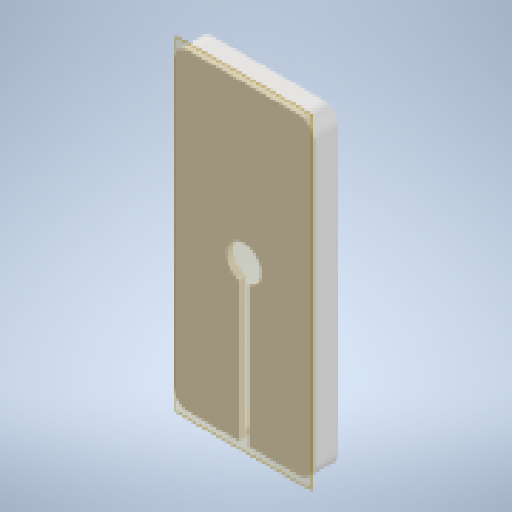
# Autodesk Inventor part: cache_batterie_1
Saved by Autodesk Inventor 2023 (Build 270158000, 158)
## iProperties
Created: 2023-03-28
Part Number: cache_batterie_1
Material: Générique
Document SubType Name: Modeling
Designer: eleves
Density: 1 g/cm^3
Appearance: Par défaut
Author: eleves
Autodesk Inventor part; units mm, degrees
ref_plane "YZ Plane" through (0, 0, 0) normal (1, 0, 0) x (0, 1, 0)
ref_plane "XZ Plane" through (0, 0, 0) normal (0, 1, 0) x (-1, 0, 0)
ref_plane "XY Plane" through (0, 0, 0) normal (0, 0, 1) x (1, 0, 0)
ref_plane "Plan de construction1" through (0, 0, 0) normal (0, 0, 1) x (1, 0, 0)
sketch "Esquisse1" plane through (0, 0, 0) normal (0, 0, 1) x (1, 0, 0)
  arc A0 (0, -82) -> (2, -84) centre (2, -82) ccw construction
  line L0 (2, -84) -> (33, -84) construction
  arc A1 (33, -84) -> (35, -82) centre (33, -82) ccw construction
  line L1 (35, -2) -> (35, -82) construction
  arc A2 (35, -2) -> (33, 0) centre (33, -2) ccw construction
  line L2 (2, 0) -> (33, 0) construction
  arc A3 (2, 0) -> (0, -2) centre (2, -2) ccw construction
  line L3 (0, -2) -> (0, -82) construction
  line L4 (2, -82) -> (33, -82) construction
  line L5 (2, -2) -> (2, -82) construction
  line L6 (2, -2) -> (33, -2) construction
  line L7 (33, -2) -> (33, -82) construction
  arc A4 (33, -84.4) -> (35.4, -82) centre (33, -82) ccw
  line L8 (33, -84.4) -> (2, -84.4)
  arc A5 (-0.4, -82) -> (2, -84.4) centre (2, -82) ccw
  line L9 (-0.4, -82) -> (-0.4, -2)
  arc A6 (2, 0.4) -> (-0.4, -2) centre (2, -2) ccw
  line L10 (2, 0.4) -> (33, 0.4)
  arc A7 (35.4, -2) -> (33, 0.4) centre (33, -2) ccw
  line L11 (35.4, -2) -> (35.4, -82)
  arc A8 (33, -86.4) -> (37.4, -82) centre (33, -82) ccw
  line L12 (33, -86.4) -> (2, -86.4)
  arc A9 (-2.4, -82) -> (2, -86.4) centre (2, -82) ccw
  line L13 (-2.4, -82) -> (-2.4, -2)
  arc A10 (2, 2.4) -> (-2.4, -2) centre (2, -2) ccw
  line L14 (2, 2.4) -> (33, 2.4)
  arc A11 (37.4, -2) -> (33, 2.4) centre (33, -2) ccw
  line L15 (37.4, -2) -> (37.4, -82)
  point P0 (0, 0)
  dimension "d0" = 0.4
  dimension "d1" = 2
  constraints: 16 end point, 16 point on circle, 8 centre point, 14 other
  measures "d0" distance between parallel lines of L1 L11
  measures "d1" distance between parallel lines of L10 L14
extrude "Extrusion1" add sketch "Esquisse1" against normal blind 2 contours L8 A5 L9 A6 L10 A7 L11 A4 | L12 A9 L13 A10 L14 A11 L15 A8
sketch "Esquisse2" plane through (0, 0, -2) normal (0, 0, -1) x (-1, 0, 0)
  line L0 (-33, -86.4) -> (-2, -86.4) projected
  arc A0 (-2, -86.4) -> (2.4, -82) centre (-2, -82) ccw projected
  line L1 (2.4, -82) -> (2.4, -2) projected
  arc A1 (2.4, -2) -> (-2, 2.4) centre (-2, -2) ccw projected
  line L2 (-2, 2.4) -> (-33, 2.4) projected
  arc A2 (-33, 2.4) -> (-37.4, -2) centre (-33, -2) ccw projected
  line L3 (-37.4, -2) -> (-37.4, -82) projected
  arc A3 (-37.4, -82) -> (-33, -86.4) centre (-33, -82) ccw projected
  line L4 (0.4, -2) -> (0.4, -82)
  arc A4 (-2, -84.4) -> (0.4, -82) centre (-2, -82) ccw
  line L5 (-2, -84.4) -> (-33, -84.4)
  arc A5 (-35.4, -82) -> (-33, -84.4) centre (-33, -82) ccw
  line L6 (-35.4, -82) -> (-35.4, -2)
  arc A6 (-33, 0.4) -> (-35.4, -2) centre (-33, -2) ccw
  line L7 (-33, 0.4) -> (-2, 0.4)
  arc A7 (0.4, -2) -> (-2, 0.4) centre (-2, -2) ccw
  point P0 (0, 0)
  dimension "d4" = 2
  constraints: 8 end point, 8 point on circle, 4 centre point, 7 other
  measures "d4" distance between parallel lines of L2 L7
extrude "Extrusion2" add sketch "Esquisse2" along normal blind 5
sketch "Esquisse3" plane through (0, 0, 0) normal (0, 0, 1) x (1, 0, 0)
  line L0 (2, -86.4) -> (33, -86.4) projected
  arc A0 (33, -86.4) -> (37.4, -82) centre (33, -82) ccw projected
  line L1 (37.4, -82) -> (37.4, -2) projected
  arc A1 (37.4, -2) -> (33, 2.4) centre (33, -2) ccw projected
  line L2 (33, 2.4) -> (2, 2.4) projected
  arc A2 (2, 2.4) -> (-2.4, -2) centre (2, -2) ccw projected
  line L3 (-2.4, -2) -> (-2.4, -82) projected
  arc A3 (-2.4, -82) -> (2, -86.4) centre (2, -82) ccw projected
  line L4 (33, -2) -> (2, -82) construction
  line L5 (2, -82) -> (33, -82) construction
  line L6 (2, -84.4) -> (33, -84.4) construction
  line L7 (2, -2) -> (33, -82) construction
  circle A4 centre (17.5, -42) radius 5
  point P0 (0, 0)
  dimension "d7" = 10
  constraints: 6 end point, 1 centre point, 1 midpoint, 1 parallel
  measures "d7" diameter of A4
extrude "Extrusion3" cut sketch "Esquisse3" against normal blind 30.25 contours A4
sketch "Esquisse4" plane through (0, 0, 0) normal (0, 0, 1) x (1, 0, 0)
  circle A0 centre (17.5, -42) radius 5 projected
  line L0 (2, -86.4) -> (33, -86.4) projected
  arc A1 (33, -86.4) -> (37.4, -82) centre (33, -82) ccw projected
  line L1 (37.4, -82) -> (37.4, -2) projected
  arc A2 (37.4, -2) -> (33, 2.4) centre (33, -2) ccw projected
  line L2 (33, 2.4) -> (2, 2.4) projected
  arc A3 (2, 2.4) -> (-2.4, -2) centre (2, -2) ccw projected
  line L3 (-2.4, -2) -> (-2.4, -82) projected
  arc A4 (-2.4, -82) -> (2, -86.4) centre (2, -82) ccw projected
  line L4 (17.5, -42) -> (19.1086, -42)
  line L5 (19.1086, -42) -> (19.1086, -46.7342)
  line L6 (17.5, -42) -> (16.1086, -42)
  line L7 (16.1086, -42) -> (16.1086, -46.8025)
  circle A5 centre (17.5, -42) radius 5 projected
  line L8 (19.1086, -46.7342) -> (19.1086, -86.4)
  line L9 (16.1086, -46.8025) -> (16.1086, -86.4)
  point P0 (0, 0)
  dimension "d11" = 3
  constraints: 12 end point, 3 point on line, 2 horizontal, 2 perpendicular, 1 point on circle, 1 vertical, 2 other
  measures "d11" distance between parallel lines of L5 L7
extrude "Extrusion4" cut sketch "Esquisse4" against normal blind 35.25 fills toward (16.1586, -66.6012) open curves L9 L7 L6 L4 L5 L8
